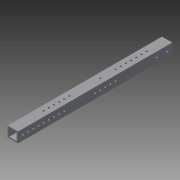
# Autodesk Inventor part: Vertical 15 in Segments (2)
Saved by Autodesk Inventor 2014 (Build 180170000, 170)
## iProperties
Created: 2014-02-24
Part Number: Vertical 15 in Segments (2)
Material: Generic
Document SubType Name: Modeling
Designer: Michael
Density: 1 g/cm^3
Appearance: Default
Author: Michael
Autodesk Inventor part; units mm, degrees
ref_plane "YZ Plane" through (0, 0, 0) normal (1, 0, 0) x (0, 1, 0)
ref_plane "XZ Plane" through (0, 0, 0) normal (0, 1, 0) x (-1, 0, 0)
ref_plane "XY Plane" through (0, 0, 0) normal (0, 0, 1) x (1, 0, 0)
sketch "Sketch1" plane through (0, 0, 0) normal (0, 0, 1) x (1, 0, 0)
  line L0 (0, 0) -> (25.4, 0)
  line L1 (25.4, 0) -> (25.4, 25.4)
  line L2 (25.4, 25.4) -> (0, 25.4)
  line L3 (0, 25.4) -> (0, 0)
  line L4 (3.175, 22.225) -> (22.225, 22.225)
  line L5 (22.225, 22.225) -> (22.225, 3.175)
  line L6 (22.225, 3.175) -> (3.175, 3.175)
  line L7 (3.175, 3.175) -> (3.175, 22.225)
  dimension "d0" = 25.4
  dimension "d1" = 25.4
  dimension "d2" = 3.175
  constraints: 16 end point, 4 parallel, 2 perpendicular, 1 horizontal, 3 other
  measures "d0" distance of L2.end L1.end
  measures "d1" distance of L1.end L0.end
  measures "d2" distance between parallel lines of L2 L4
extrude "Extrusion1" add sketch "Sketch1" along normal blind 381
sketch "Sketch2" plane through (25.4, 0, 0) normal (1, 0, 0) x (0, 0, -1)
  line L0 (0, 0) -> (0, 25.4) projected
  line L1 (-381, 0) -> (-381, 25.4) projected
  line L2 (0, 0) -> (-381, 0) projected
  circle A0 centre (-368.3, 12.7) radius 2.0701
  circle A1 centre (-355.6, 12.7) radius 2.0701
  circle A2 centre (-342.9, 12.7) radius 2.0701
  circle A3 centre (-330.2, 12.7) radius 2.0701
  circle A4 centre (-317.5, 12.7) radius 2.0701
  circle A5 centre (-304.8, 12.7) radius 2.0701
  circle A6 centre (-292.1, 12.7) radius 2.0701
  circle A7 centre (-279.4, 12.7) radius 2.0701
  circle A8 centre (-266.7, 12.7) radius 2.0701
  circle A9 centre (-190.5, 12.7) radius 2.0701
  circle A10 centre (-177.8, 12.7) radius 2.0701
  circle A11 centre (-165.1, 12.7) radius 2.0701
  circle A12 centre (-152.4, 12.7) radius 2.0701
  circle A13 centre (-139.7, 12.7) radius 2.0701
  circle A14 centre (-12.7, 12.7) radius 2.0701
  circle A15 centre (-38.1, 12.7) radius 2.0701
  dimension "d5" = 4.1402
  dimension "d6" = 12.7
  dimension "d7" = 12.7
  dimension "d10" = 12.7
  dimension "d15" = 76.2
  dimension "d16" = 12.7
  dimension "d19" = 12.7
  dimension "d24" = 12.7
  dimension "d25" = 12.7
  dimension "d28" = 25.4
  constraints: 16 centre point, 3 horizontal, 2 equal radius, 26 other
  measures "d5" diameter of A0
  measures "d6" distance from line of L2 A0.centre
  measures "d7" distance from line of L1 A0.centre
  measures "d10" distance of A0.centre A1.centre
  measures "d15" distance of A9.centre A8.centre
  measures "d16" distance from line of A9.centre L2
  measures "d19" distance of A9.centre A10.centre
  measures "d24" distance from line of L0 A14.centre
  measures "d25" distance from line of L2 A14.centre
  measures "d28" distance of A14.centre A15.centre
extrude "Extrusion2" cut sketch "Sketch2" against normal blind 381
sketch "Sketch3" plane through (0, 25.4, 0) normal (0, 1, 0) x (1, 0, 0)
  line L0 (25.4, 0) -> (0, 0) projected
  line L1 (25.4, -381) -> (0, -381) projected
  line L2 (25.4, 0) -> (25.4, -381) projected
  circle A0 centre (12.7, -304.8) radius 2.0701
  circle A1 centre (12.7, -292.1) radius 2.0701
  circle A2 centre (12.7, -279.4) radius 2.0701
  circle A3 centre (12.7, -266.7) radius 2.0701
  circle A4 centre (12.7, -254) radius 2.0701
  circle A5 centre (12.7, -241.3) radius 2.0701
  circle A6 centre (12.7, -50.8) radius 2.0701
  circle A7 centre (12.7, -63.5) radius 2.0701
  circle A8 centre (12.7, -76.2) radius 2.0701
  circle A9 centre (12.7, -88.9) radius 2.0701
  circle A10 centre (12.7, -101.6) radius 2.0701
  circle A11 centre (12.7, -114.3) radius 2.0701
  circle A12 centre (12.7, -127) radius 2.0701
  circle A13 centre (12.7, -165.1) radius 2.0701
  dimension "d35" = 4.1402
  dimension "d36" = 76.2
  dimension "d37" = 12.7
  dimension "d40" = 12.7
  dimension "d45" = 50.8
  dimension "d46" = 12.7
  dimension "d49" = 12.7
  dimension "d54" = 38.1
  dimension "d55" = 12.7
  constraints: 14 centre point, 2 equal radius, 2 vertical, 22 other
  measures "d35" diameter of A0
  measures "d36" distance from line of L1 A0.centre
  measures "d37" distance from line of L2 A0.centre
  measures "d40" distance of A0.centre A1.centre
  measures "d45" distance from line of L0 A6.centre
  measures "d46" distance from line of L2 A6.centre
  measures "d49" distance of A6.centre A7.centre
  measures "d54" distance of A13.centre A12.centre
  measures "d55" distance from line of L2 A13.centre
extrude "Extrusion3" cut sketch "Sketch3" against normal blind 381
body "Solid1"
